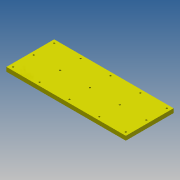
# Autodesk Inventor part: CNC Assembly
Saved by Autodesk Inventor 2015 (Build 190159000, 159)
## iProperties
Created: 2014-10-08
Part Number: CNC Assembly
Material: PET Plastic
Document SubType Name: Modeling
Designer: jdyne
Density: 1.541 g/cm^3
Appearance: Smooth - Yellow
Author: jdyne
Autodesk Inventor part; units mm, degrees
ref_plane "YZ Plane" through (0, 0, 0) normal (1, 0, 0) x (0, 1, 0)
ref_plane "XZ Plane" through (0, 0, 0) normal (0, 1, 0) x (-1, 0, 0)
ref_plane "XY Plane" through (0, 0, 0) normal (0, 0, 1) x (1, 0, 0)
sketch "Sketch1" plane through (0, 0, 0) normal (0, 0, 1) x (1, 0, 0)
  line L0 (-142.5, 57) -> (142.5, 57)
  line L1 (142.5, 57) -> (142.5, -57)
  line L2 (142.5, -57) -> (-142.5, -57)
  line L3 (-142.5, -57) -> (-142.5, 57)
  point P0 (0, 0)
  dimension "d0" = 114
  dimension "d1" = 285
  dimension "d2" = 57
  dimension "d3" = 142.5
  constraints: 8 end point, 2 parallel, 1 horizontal, 1 perpendicular
  measures "d0" distance between parallel lines of L2 L0
  measures "d1" distance of L0.start L0.end
  measures "d2" distance from line of point (0, 0) L0
  measures "d3" distance from line of point (0, 0) L3
extrude "Extrusion1" add sketch "Sketch1" along normal blind 10
sketch "Sketch2" plane through (0, 0, 10) normal (0, 0, 1) x (1, 0, 0)
  line L0 (142.5, 57) -> (-142.5, 57) projected
  line L1 (-142.5, 57) -> (-142.5, -57) projected
  line L2 (-142.5, -57) -> (142.5, -57) projected
  line L3 (142.5, -57) -> (142.5, 57) projected
  point P0 (0, 0)
  point P1 (-134.5, 49)
  point P2 (-134.5, -49)
  point P3 (134.5, -49)
  point P4 (134.5, 49)
  point P5 (71.25, 49)
  point P6 (-71.25, 49)
  point P7 (-71.25, -49)
  point P8 (71.25, -49)
  point P9 (-71.25, 0)
  point P10 (0, 0)
  point P11 (71.25, 0)
  point P12 (0, 49)
  point P13 (0, -49)
  point P14 (-134.5, 0)
  point P15 (134.5, 0)
  dimension "d6" = 8
  dimension "d7" = 8
  dimension "d8" = 8
  dimension "d9" = 8
  dimension "d13" = 71.25
  dimension "d14" = 71.25
  dimension "d15" = 71.25
  dimension "d16" = 71.25
  constraints: 12 horizontal alignment, 10 vertical alignment, 1 coincident
  measures "d6" distance from line of point (-134.5, 49) L1
  measures "d7" distance from line of L3 point (134.5, 49)
  measures "d8" distance from line of L2 point (134.5, -49)
  measures "d9" distance from line of L0 point (134.5, 49)
  measures "d13" distance from line of point (-71.25, 0) L1
  measures "d14" distance of point (0, 0) point (-71.25, 0)
  measures "d15" distance from line of L3 point (71.25, 0)
  measures "d16" distance of point (0, 0) point (71.25, 0)
hole "Hole1" at (-134.5, 49, 10) at (-134.5, -49, 10) at (134.5, -49, 10) at (134.5, 49, 10) at (71.25, 49, 10) at (-71.25, 49, 10) at (-71.25, -49, 10) at (71.25, -49, 10) at (-71.25, 0, 10) at (0, 0, 10) at (71.25, 0, 10) at (0, 49, 10) at (0, -49, 10) at (-134.5, 0, 10) at (134.5, 0, 10) direction (0, 0, -1) diameter 4 end through all
equation "\"d2\" = 0.5 * d0"
equation "\"d3\" = 0.5 * d1"
equation "\"d13\" = d14"
equation "\"d15\" = d14"
body "Solid1"
